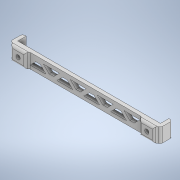
# Autodesk Inventor part: jetnxmount
Saved by Autodesk Inventor 2022 (Build 260153000, 153)
## iProperties
Created: 2022-02-08
Part Number: jetnxmount
Material: Generic
Document SubType Name: Modeling
Designer: ARRF
Density: 1 g/cm^3
Appearance: Default
Author: ARRF
Autodesk Inventor part; units mm, degrees
ref_plane "YZ Plane" through (0, 0, 0) normal (1, 0, 0) x (0, 1, 0)
ref_plane "XZ Plane" through (0, 0, 0) normal (0, 1, 0) x (-1, 0, 0)
ref_plane "XY Plane" through (0, 0, 0) normal (0, 0, 1) x (1, 0, 0)
sketch "Sketch1" plane through (0, 0, 0) normal (0, 0, 1) x (1, 0, 0)
  line L0 (-59.5, -6) -> (59.5, -6)
  line L1 (59.5, -6) -> (59.5, 6)
  line L2 (59.5, 6) -> (-59.5, 6)
  line L3 (-59.5, 6) -> (-59.5, -6)
  line L4 (-59.5, -6) -> (59.5, 6) construction
  line L5 (59.5, -6) -> (-59.5, 6) construction
  point P0 (0, 0)
  dimension "d0" = 119
  dimension "d1" = 12
  constraints: 12 end point, 2 midpoint, 2 parallel, 1 horizontal, 1 perpendicular
  measures "d0" distance of L2.end L1.end
  measures "d1" distance of L1.end L0.end
extrude "Extrusion1" add sketch "Sketch1" along normal blind 3
sketch "Sketch2" plane through (-59.5, -6, 0) normal (-1, 0, 0) x (0, 0, 1)
  line L0 (3, 0) -> (3, 12) projected
  line L1 (0, 0) -> (3, 0) projected
  line L2 (3, 12) -> (3, 0)
  line L3 (3, 0) -> (-7, 0)
  line L4 (-7, 0) -> (-7, 12)
  line L5 (-7, 12) -> (3, 12)
  point P0 (0, 6)
  dimension "d4" = 10
  constraints: 8 end point, 2 parallel, 2 perpendicular
  measures "d4" distance of L0.start L3.end
extrude "Extrusion2" add sketch "Sketch2" along normal blind 3
sketch "Sketch3" plane through (0, 0, 0) normal (0, 0, -1) x (-1, 0, 0)
  circle A0 centre (53.7, 0) radius 3.1
  point P0 (0, 0)
  dimension "d7" = 6.2
  dimension "d12" = 53.7
  constraints: 1 centre point
  measures "d7" diameter of A0
  measures "d12" distance of A0.centre point (0, 0)
extrude "Extrusion3" cut sketch "Sketch3" against normal blind 3.5
sketch "Sketch4" plane through (0, 0, 3) normal (0, 0, 1) x (1, 0, 0)
  line L0 (-62.5, -6) -> (-62.5, 6)
  line L1 (-47.5569, 6) -> (-59.8431, 6)
  line L2 (-59.8431, 6) -> (-59.8431, -6)
  line L3 (-59.8431, -6) -> (-47.5569, -6)
  line L4 (-47.5569, -6) -> (-47.5569, 6)
  line L5 (-47.5569, 6) -> (-59.8431, -6) construction
  line L6 (-59.8431, 6) -> (-47.5569, -6) construction
  point P0 (0, 0)
  point P1 (-53.7, 0)
  dimension "d16" = 53.7
  constraints: 14 end point, 2 midpoint, 2 parallel, 1 horizontal, 1 perpendicular
  measures "d16" distance of point (0, 0) point (-53.7, 0)
extrude "Extrusion4" add sketch "Sketch4" along normal blind 2.5
sketch "Sketch5" plane through (-53.7, 0, 3) normal (0, 0, -1) x (-1, 0, 0)
  circle A0 centre (0, 0) radius 3.1 projected
  circle A1 centre (0, 0) radius 1.75
  point P0 (-53.7, 0)
  dimension "d13" = 3.5
  constraints: 1 centre point, 1 coincident
  measures "d13" diameter of A1
extrude "Extrusion5" cut sketch "Sketch5" against normal blind 2.5 contours A1
fillet "Fillet1" radius 2 8 edges at (-53.7, -6, 5.5) (-59.8431, 0, 5.5) (-62.5, 0, 3) (-59.8431, 0, 3) (-53.7, 6, 5.5) (-47.5569, 0, 5.5) (-47.5569, 0, 3) (-62.5, 0, -7)
mirror "Mirror1" about plane through (0, 0, 0) normal (1, 0, 0) of "Extrusion2", "Extrusion3", "Extrusion4", "Extrusion5", "Fillet1"
sketch "Sketch6" plane through (0, 0, 0) normal (0, 0, -1) x (-1, 0, 0)
  circle A0 centre (-53.7, 0) radius 3.1 projected
  circle A1 centre (53.7, 0) radius 3.1 projected
  line L0 (-59.5, -6) -> (-59.5, 6) projected
  line L1 (59.5, -6) -> (-59.5, -6) projected
  line L2 (59.5, 6) -> (59.5, -6) projected
  line L3 (-59.5, 6) -> (59.5, 6) projected
  line L4 (56.6035, 3.1035) -> (56.6035, -3.1035)
  line L5 (56.6035, -3.1035) -> (-56.6035, -3.1035)
  line L6 (-56.6035, -3.1035) -> (-56.6035, 3.1035)
  line L7 (-56.6035, 3.1035) -> (56.6035, 3.1035)
  line L8 (-47.5569, 3.1035) -> (-41.3499, -3.1035)
  line L9 (-47.5569, 3.1035) -> (-38.7788, 3.1035) construction
  line L10 (-41.3499, -3.1035) -> (-36.3499, -3.1035)
  line L11 (-36.3499, -3.1035) -> (-30.1429, 3.1035)
  line L12 (-30.1429, 3.1035) -> (-25.1429, 3.1035)
  line L13 (-25.1429, 3.1035) -> (-18.9359, -3.1035)
  line L14 (-18.9359, -3.1035) -> (-13.9359, -3.1035)
  line L15 (-13.9359, -3.1035) -> (-7.7289, 3.1035)
  line L16 (-7.7289, 3.1035) -> (-2.7289, 3.1035)
  line L17 (-2.7289, 3.1035) -> (3.4781, -3.1035)
  line L18 (3.4781, -3.1035) -> (8.4781, -3.1035)
  line L19 (8.4781, -3.1035) -> (14.6851, 3.1035)
  line L20 (14.6851, 3.1035) -> (19.6851, 3.1035)
  line L21 (19.6851, 3.1035) -> (25.8921, -3.1035)
  line L22 (25.8921, -3.1035) -> (30.8921, -3.1035)
  line L23 (30.8921, -3.1035) -> (37.0991, 3.1035)
  line L24 (37.0991, 3.1035) -> (42.0991, 3.1035)
  line L25 (42.0991, 3.1035) -> (48.3061, -3.1035)
  line L26 (47.2455, -4.1642) -> (41.4778, 1.6035)
  line L27 (41.4778, 1.6035) -> (37.7205, 1.6035)
  line L28 (37.7205, 1.6035) -> (31.5135, -4.6035)
  line L29 (31.5135, -4.6035) -> (25.2708, -4.6035)
  line L30 (25.2708, -4.6035) -> (19.0638, 1.6035)
  line L31 (19.0638, 1.6035) -> (15.3065, 1.6035)
  line L32 (15.3065, 1.6035) -> (9.0995, -4.6035)
  line L33 (9.0995, -4.6035) -> (2.8568, -4.6035)
  line L34 (2.8568, -4.6035) -> (-3.3502, 1.6035)
  line L35 (-3.3502, 1.6035) -> (-7.1075, 1.6035)
  line L36 (-7.1075, 1.6035) -> (-13.3145, -4.6035)
  line L37 (-13.3145, -4.6035) -> (-19.5572, -4.6035)
  line L38 (-19.5572, -4.6035) -> (-25.7642, 1.6035)
  line L39 (-25.7642, 1.6035) -> (-29.5215, 1.6035)
  line L40 (-29.5215, 1.6035) -> (-35.7285, -4.6035)
  line L41 (-35.7285, -4.6035) -> (-41.9712, -4.6035)
  line L42 (-41.9712, -4.6035) -> (-51.1782, 4.6035)
  line L43 (-51.1782, 4.6035) -> (-38.7788, 4.6035)
  line L44 (49.3668, -2.0428) -> (42.7205, 4.6035)
  line L45 (42.7205, 4.6035) -> (36.4778, 4.6035)
  line L46 (36.4778, 4.6035) -> (30.2708, -1.6035)
  line L47 (30.2708, -1.6035) -> (26.5135, -1.6035)
  line L48 (26.5135, -1.6035) -> (20.3065, 4.6035)
  line L49 (20.3065, 4.6035) -> (14.0638, 4.6035)
  line L50 (14.0638, 4.6035) -> (7.8568, -1.6035)
  line L51 (7.8568, -1.6035) -> (4.0995, -1.6035)
  line L52 (4.0995, -1.6035) -> (-2.1075, 4.6035)
  line L53 (-2.1075, 4.6035) -> (-8.3502, 4.6035)
  line L54 (-8.3502, 4.6035) -> (-14.5572, -1.6035)
  line L55 (-14.5572, -1.6035) -> (-18.3145, -1.6035)
  line L56 (-18.3145, -1.6035) -> (-24.5215, 4.6035)
  line L57 (-24.5215, 4.6035) -> (-30.7642, 4.6035)
  line L58 (-30.7642, 4.6035) -> (-36.9712, -1.6035)
  line L59 (-36.9712, -1.6035) -> (-40.7285, -1.6035)
  line L60 (-40.7285, -1.6035) -> (-43.9355, 1.6035)
  line L61 (-43.9355, 1.6035) -> (-38.7788, 1.6035)
  line L62 (-43.9355, 1.6035) -> (-45.5569, 3.1035)
  line L63 (-45.5569, 6) -> (-45.5569, -6) projected
  line L64 (49.3668, -2.0428) -> (50.5132, -3.1035)
  point P0 (0, 0)
  point P1 (34.9778, 3.1035)
  point P2 (21.8065, 3.1035)
  point P3 (33.0135, -3.1035)
  point P4 (46.1848, -3.1035)
  point P5 (-34.2285, -3.1035)
  point P6 (-21.0572, -3.1035)
  point P7 (-11.8145, -3.1035)
  point P8 (1.3568, -3.1035)
  point P9 (10.5995, -3.1035)
  point P10 (23.7708, -3.1035)
  point P11 (12.5638, 3.1035)
  point P12 (-0.6075, 3.1035)
  point P13 (-9.8502, 3.1035)
  point P14 (-23.0215, 3.1035)
  point P15 (-32.2642, 3.1035)
  dimension "d18" = 45
  dimension "d19" = 5
  dimension "d20" = 5
  dimension "d21" = 5
  dimension "d22" = 5
  dimension "d23" = 5
  dimension "d24" = 5
  dimension "d25" = 5
  dimension "d26" = 5
  dimension "d27" = 1.5
  dimension "d28" = 1.5
  constraints: 116 end point, 21 perpendicular, 2 point on line, 1 equal length, 1 horizontal, 1 parallel, 62 other
  measures "d18" angle of L8 L9
  measures "d19" distance of L8.end L10.end
  measures "d20" distance of L11.end L12.end
  measures "d21" distance of L13.end L14.end
  measures "d22" distance of L15.end L16.end
  measures "d23" distance of L17.end L18.end
  measures "d24" distance of L19.end L20.end
  measures "d25" distance of L21.end L22.end
  measures "d26" distance of L23.end L24.end
  measures "d27" distance between parallel lines of L8 L42
  measures "d28" distance between parallel lines of L8 L60
extrude "Extrusion6" cut sketch "Sketch6" against normal through all contours L7 L58 L59 L60 L62 | L40 L39 L38 L5 | L7 L54 L55 L56 | L36 L35 L34 L5 | L7 L50 L51 L52 | L32 L31 L30 L5 | L7 L46 L47 L48 | L28 L27 L26 L5
body "Solid1"
